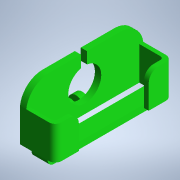
# Autodesk Inventor part: cam_hold_logitech
Saved by Autodesk Inventor 2022 (Build 260153000, 153)
## iProperties
Created: 2022-10-11
Part Number: cam_hold_logitech
Material: Типовые
Document SubType Name: Modeling
Designer: korsh624
Density: 1 g/cm^3
Appearance: Темно-зеленый
Author: korsh624
Autodesk Inventor part; units mm, degrees
ref_plane "YZ Plane" through (0, 0, 0) normal (1, 0, 0) x (0, 1, 0)
ref_plane "XZ Plane" through (0, 0, 0) normal (0, 1, 0) x (-1, 0, 0)
ref_plane "XY Plane" through (0, 0, 0) normal (0, 0, 1) x (1, 0, 0)
sketch "Эскиз1" plane through (0, 0, 0) normal (0, 0, 1) x (1, 0, 0)
  arc A0 (-3.5681, 4.8905) -> (-4.8473, 3.794) centre (-3.4, 3.4) ccw projected
  circle A1 centre (-3.4, 3.4) radius 1.5
  arc A2 (0.4144, 4.9) -> (0.4144, 1.9) centre (-3.4, 3.4) ccw
  line L0 (0.4144, 4.9) -> (0.4144, 1.9)
  point P0 (0, 0)
  point P1 (-4.8473, 3.794)
  point P2 (-3.5681, 4.8905)
  constraints: 2 centre point, 2 coincident, 2 end point, 2 point on circle, 1 concentric, 1 vertical
extrude "Выдавливание1" add sketch "Эскиз1" along normal blind 4
sketch "Эскиз2" plane through (0.4144, 1.9, 0) normal (1, 0, 0) x (0, 0, -1)
  line L0 (0, 0) -> (0, 3) projected
  line L1 (0, 3) -> (-4, 3) projected
  line L2 (-4, 0) -> (-4, 3) projected
  line L3 (0, 0) -> (-4, 0) projected
  line L4 (0, 3) -> (-4, 3) projected
  line L5 (-4, 3) -> (7.5, 3)
  line L6 (7.5, 3) -> (7.5, 0)
  line L7 (7.5, 0) -> (-4, 0)
  line L8 (-4, 0) -> (-4, 3)
  point P0 (0, -1.9)
  point P1 (3, 1.9)
  dimension "d2" = 4
  dimension "d3" = 4.5
  constraints: 8 end point, 2 parallel, 1 horizontal, 1 perpendicular, 1 point on line, 1 other
  measures "d2" distance between parallel lines of L0 L2
  measures "d3" distance from line of point (3, 1.9) L6
extrude "Выдавливание2" add sketch "Эскиз2" along normal blind 3
sketch "Эскиз3" plane through (0.4144, 1.9, -7.5) normal (0, 0, -1) x (-1, 0, 0)
  line L0 (0, 0) -> (0, 3) projected
  arc A0 (0, 0) -> (0, 3) centre (3.8144, 1.5) ccw projected
  circle A1 centre (3.8144, 1.5) radius 1.5 projected
  point P0 (0.4144, -1.9)
extrude "Выдавливание3" add sketch "Эскиз3" against normal blind 4
sketch "Эскиз4" plane through (3.4144, 1.9, 0) normal (1, 0, 0) x (0, 0, -1)
  line L0 (6.3383, 0) -> (-1.6617, 0) projected
  line L1 (39.5883, 0) -> (-34.9117, 0)
  line L2 (-34.9117, 0) -> (-34.9117, 21.3)
  line L3 (-21.0745, 33.9845) -> (25.7512, 33.9845)
  line L4 (39.5883, 21.3002) -> (39.5883, 0)
  line L5 (-31.9117, 21.3) -> (-31.9117, 4.3) projected
  line L6 (36.5883, 4.3) -> (36.5883, 21.3) projected
  line L7 (24.5883, 33.3) -> (-19.9117, 33.3) projected
  arc A0 (-19.9117, 33.9845) -> (-34.9117, 21.3) centre (-20.4931, 19.4607) ccw
  circle A1 centre (2.3383, 16.3) radius 0.9967 projected
  line L8 (2.3383, 16.3) -> (2.3383, 42.847) construction
  arc A2 (39.5883, 21.3) -> (24.5883, 33.9845) centre (25.1697, 19.4607) ccw
  point P0 (0, -1.9)
  point P1 (-1.6617, 0)
  dimension "d8" = 3
  dimension "d9" = 3
  constraints: 10 end point, 7 point on circle, 3 symmetric about line, 2 centre point, 2 parallel, 1 horizontal, 1 perpendicular, 1 point on line, 1 vertical, 1 other
  measures "d8" distance between parallel lines of L6 L4
  measures "d9" distance between parallel lines of L2 L5
extrude "Выдавливание4" add sketch "Эскиз4" against normal blind 4 contours L0 L1 L2 A0 L3 A2 L4
sketch "Эскиз5" plane through (-0.5856, 1.9, 0) normal (-1, 0, 0) x (0, 0, 1)
  arc A0 (-10.3389, 9.5) -> (5.6623, 9.5) centre (-2.3383, 16.3) ccw projected
  circle A1 centre (-2.3383, 16.3) radius 0.9967 projected
  circle A2 centre (-2.3383, 16.3) radius 10.5
  point P0 (0, -1.9)
  point P1 (5.6623, 9.5)
  point P2 (-10.3389, 9.5)
  constraints: 1 centre point, 1 coincident, 1 concentric
extrude "Выдавливание5" cut sketch "Эскиз5" against normal blind 4
sketch "Эскиз6" plane through (3.4144, 1.9, 0) normal (1, 0, 0) x (0, 0, -1)
  circle A0 centre (2.3383, 16.3) radius 10.5 projected
  line L0 (-34.9117, 0) -> (39.5883, 0) projected
  line L1 (39.5883, 0) -> (39.5883, 21.3002) projected
  arc A1 (39.5883, 21.3002) -> (25.7512, 33.9845) centre (25.1697, 19.4607) ccw projected
  line L2 (25.7512, 33.9845) -> (-21.0745, 33.9845) projected
  arc A2 (-21.0745, 33.9845) -> (-34.9117, 21.3) centre (-20.4931, 19.4607) ccw projected
  line L3 (-34.9117, 21.3) -> (-34.9117, 0) projected
  line L4 (-34.9117, 0) -> (-32.4117, 0)
  line L5 (-32.4117, 0) -> (-32.4117, 21.3)
  line L6 (-32.4117, 21.3) -> (-34.9117, 21.3)
  line L7 (-34.9117, 21.3) -> (-34.9117, 0)
  line L8 (39.5883, 0) -> (39.5883, 21.3002) projected
  line L9 (39.5883, 0) -> (37.0883, 0)
  line L10 (37.0883, 0) -> (37.0883, 21.3)
  line L11 (37.0883, 21.3) -> (39.5883, 21.3)
  line L12 (39.5883, 21.3) -> (39.5883, 0)
  point P0 (0, -1.9)
  dimension "d14" = 2.5
  dimension "d15" = 2.5
  constraints: 16 end point, 4 parallel, 2 horizontal, 2 perpendicular, 1 point on line
  measures "d14" distance of L6.end L5.end
  measures "d15" distance of L10.end L11.end
extrude "Выдавливание6" add sketch "Эскиз6" along normal blind 15.5 contours L3 L6 L5 L0 | L10 L11 L1 L0
sketch "Эскиз7" plane through (-0.5856, 1.9, 0) normal (-1, 0, 0) x (0, 0, 1)
  circle A0 centre (-2.3383, 16.3) radius 10.5 projected
  line L0 (-3.82, 35.4662) -> (0, 35.4662)
  line L1 (0, 35.4662) -> (0, 24.6625)
  line L2 (0, 24.6625) -> (-3.82, 24.6625)
  line L3 (-3.82, 24.6625) -> (-3.82, 35.4662)
  point P0 (0, -1.9)
  point P1 (-3.82, 26.6949)
  point P2 (0, 26.5363)
  constraints: 8 end point, 2 parallel, 1 horizontal, 1 perpendicular
extrude "Выдавливание7" cut sketch "Эскиз7" against normal blind 15.5 contours A0 L3 L0 L1
sketch "Эскиз8" plane through (0.4144, 1.9, 0) normal (0, -1, 0) x (1, 0, 0)
  line L0 (3, 32.4117) -> (18.5, 32.4117) projected
  line L1 (3, -37.0883) -> (18.5, -37.0883) projected
  line L2 (16.6252, 32.4117) -> (6.3462, 32.4117)
  line L3 (6.3462, 32.4117) -> (6.3462, -37.0883)
  line L4 (6.3462, -37.0883) -> (16.6252, -37.0883)
  line L5 (16.6252, -37.0883) -> (16.6252, 32.4117)
  line L6 (18.5, 34.9117) -> (-1, 34.9117) projected
  line L7 (16.6252, 34.9117) -> (6.3462, 34.9117)
  line L8 (6.3462, 34.9117) -> (6.3462, 32.4117)
  line L9 (6.3462, 32.4117) -> (16.6252, 32.4117)
  line L10 (16.6252, 32.4117) -> (16.6252, 34.9117)
  line L11 (-1, -39.5883) -> (18.5, -39.5883) projected
  line L12 (16.6252, -37.0883) -> (6.3462, -37.0883)
  line L13 (6.3462, -37.0883) -> (6.3462, -39.5883)
  line L14 (6.3462, -39.5883) -> (16.6252, -39.5883)
  line L15 (16.6252, -39.5883) -> (16.6252, -37.0883)
  point P0 (-0.4144, 0)
  point P1 (6.3462, -37.0883)
  constraints: 24 end point, 6 parallel, 6 point on line, 3 horizontal, 3 perpendicular
extrude "Выдавливание8" add sketch "Эскиз8" along normal blind 4
fillet "Сопряжение1" radius 4 2 edges at (11.9001, -2.1, -39.5883) (11.9001, -2.1, 34.9117)
sketch "Эскиз9" plane through (18.9144, 1.9, -39.5883) normal (0, -1, 0) x (1, 0, 0)
  line L0 (-15.5, 74.5) -> (0, 74.5) projected
  line L1 (0, 74.5) -> (3, 74.5)
  line L2 (3, 74.5) -> (3, 59.5)
  line L3 (3, 59.5) -> (0, 59.5)
  line L4 (0, 59.5) -> (0, 74.5)
  line L5 (0, 2.5) -> (0, 0) projected
  line L6 (0, 0) -> (3, 0)
  line L7 (3, 0) -> (3, 15)
  line L8 (3, 15) -> (0, 15)
  line L9 (0, 15) -> (0, 0)
  point P0 (-18.9144, 39.5883)
  dimension "d23" = 3
  dimension "d24" = 15
  dimension "d25" = 15
  constraints: 16 end point, 4 parallel, 2 horizontal, 2 perpendicular, 1 point on line
  measures "d23" distance of L2.end L3.end
  measures "d24" distance of L1.end L2.end
  measures "d25" distance of L7.end L6.end
extrude "Выдавливание9" add sketch "Эскиз9" against normal blind 21.3
fillet "Сопряжение2" radius 4 2 edges at (21.9144, 12.55, -39.5883) (21.9144, 12.55, 34.9117)
fillet "Сопряжение3" radius 2 2 edges at (18.9144, 12.55, 32.4117) (18.9144, 12.55, -37.0883)
fillet "Сопряжение4" radius 6 2 edges at (20.4144, 23.2, 19.9117) (20.4144, 23.2, -24.5883)
sketch "Эскиз10" plane through (0.4144, 1.9, -7.5) normal (0, 0, -1) x (-1, 0, 0)
  circle A0 centre (3.8144, 1.5) radius 1.5 projected
  arc A1 (0, 0) -> (1, 4.4797) centre (3.8144, 1.5) ccw projected
  arc A2 (1, -2.6327) -> (1, 5.6327) centre (3.8144, 1.5) ccw
  line L0 (1, 0) -> (1, 21.3) projected
  line L1 (1, 6.5) -> (1, -2.6327)
  point P0 (0.4144, -1.9)
  point P1 (1, -1.4797)
  dimension "d31" = 10
  constraints: 2 end point, 2 point on circle, 2 point on line, 1 centre point, 1 coincident, 1 collinear
  measures "d31" diameter of A2
extrude "Выдавливание10" add sketch "Эскиз10" against normal blind 4 contours A1 L0 A2 L1
sketch "Эскиз11" plane through (0, 0, 4) normal (0, 0, 1) x (1, 0, 0)
  arc A0 (-0.5856, 7.5327) -> (-0.5856, -0.7327) centre (-3.4, 3.4) ccw projected
  circle A1 centre (-3.4, 3.4) radius 1.5 projected
  circle A2 centre (-3.4, 3.4) radius 5
  line L0 (-0.5856, 1.9) -> (-0.5856, 7.5327) projected
  line L1 (-0.5856, 7.5327) -> (-0.5856, -0.7327)
  circle A3 centre (-3.4, 3.4) radius 1.5 projected
  line L2 (0.4144, 1.9) -> (-0.5856, 1.9) projected
  line L3 (-0.5856, 1.9) -> (-0.5856, 6.3797) projected
  arc A4 (-0.5856, 6.3797) -> (0.4144, 1.9) centre (-3.4, 3.4) ccw projected
  point P0 (0, 0)
  point P1 (-0.5856, 0.4203)
  constraints: 2 end point, 1 coincident, 1 vertical, 3 other
extrude "Выдавливание11" add sketch "Эскиз11" against normal blind 4 contours L0 A4 L1 A0
